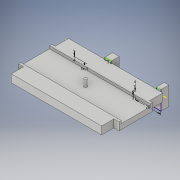
# Autodesk Inventor part: kotelon yläosa
Saved by Autodesk Inventor 2019 (Build 230136000, 136)
## iProperties
Created: 2018-07-24
Part Number: kotelon yläosa
Material: Generic
Document SubType Name: Modeling
Designer: OMISTAJA
Density: 1 g/cm^3
Appearance: Default
Author: OMISTAJA
## iProperties of the stored document kotelon yläosa_3DPrint.ipt
Created: 2018-07-24
Part Number: kotelon yläosa_3DPrint
Material: Generic
Document SubType Name: Modeling
Designer: OMISTAJA
Density: 1 g/cm^3
Appearance: Default
Author: OMISTAJA
Autodesk Inventor part; units mm, degrees
ref_plane "YZ Plane" through (0, 0, 0) normal (1, 0, 0) x (0, 1, 0)
ref_plane "XZ Plane" through (0, 0, 0) normal (0, 1, 0) x (-1, 0, 0)
ref_plane "XY Plane" through (0, 0, 0) normal (0, 0, 1) x (1, 0, 0)
sketch "Sketch1" plane through (0, 0, 0) normal (0, 1, 0) x (-1, 0, 0)
  line L0 (-36.5556, -23.5) -> (36.5556, -23.5)
  line L1 (35, 22.5) -> (-35, 22.5)
  line L2 (-36.5556, -23.5) -> (35, 22.5) construction
  line L3 (36.5556, -23.5) -> (-35, 22.5) construction
  line L4 (-39, 0) -> (-39, -11)
  line L5 (-39, -11) -> (-39, 11)
  line L6 (39, -11) -> (39, 11)
  line L7 (-39, -11) -> (-39, -13)
  line L8 (-39, -13) -> (-36.5556, -13)
  line L9 (-39, 11) -> (-39, 13)
  line L10 (-39, 13) -> (-35, 13)
  line L11 (39, -11) -> (39, -13)
  line L12 (39, -13) -> (36.5556, -13)
  line L13 (39, 11) -> (39, 13)
  line L14 (39, 13) -> (35, 13)
  line L15 (-30.788, 17.5) -> (31, 17.5)
  line L16 (31, 17.5) -> (31, -18.5)
  line L17 (31, -18.5) -> (-30.788, -18.5)
  line L18 (-30.788, -18.5) -> (-30.788, 17.5)
  line L19 (-30.788, 17.5) -> (31, -18.5) construction
  line L20 (31, 17.5) -> (-30.788, -18.5) construction
  line L21 (36.5556, -23.5) -> (36.5556, -13)
  line L22 (35, 13) -> (35, 22.5)
  line L23 (-35, 22.5) -> (-35, 13)
  line L24 (-36.5556, -13) -> (-36.5556, -23.5)
  circle A0 centre (0, 0) radius 1.25
  dimension "d133" = 2.5
  dimension "d169" = 36
  dimension "d170" = 4
  dimension "d171" = 5
  dimension "d180" = 46
  constraints: 50 end point, 11 perpendicular, 7 parallel, 4 point on line, 3 vertical, 2 horizontal, 1 centre point, 1 coincident
  measures "d133" diameter of A0
  measures "d169" distance between parallel lines of L17 L15
  measures "d170" distance between parallel lines of L22 L16
  measures "d171" distance between parallel lines of L0 L17
  measures "d180" distance between parallel lines of L0 L1
extrude "Extrusion39" add sketch "Sketch1" along normal blind 6 contours L24 L8 L7 L4 L5 L9 L10 L23 L1 L22 L14 L13 L6 L11 L12 L21 L0
extrude "Extrusion40" add sketch "Sketch1" against normal blind 2 contours L15 L16 L17 L18
extrude "Extrusion41" add sketch "Sketch1" along normal blind 6 contours L15 L16 L17 L18
extrude "Extrusion42" add sketch "Sketch1" along normal blind 9 contours A0
sketch "Sketch30" plane through (0, 6, 0) normal (0, 1, 0) x (1, 0, 0)
  line L0 (-39, -11.25) -> (39, -11.25)
  line L1 (39, -11.25) -> (39, 11.25)
  line L2 (39, 11.25) -> (-39, 11.25)
  line L3 (-39, 11.25) -> (-39, -11.25)
  circle A0 centre (0, 0) radius 1.25 projected
  line L4 (-39, -11.25) -> (39, 11.25) construction
  line L5 (39, -11.25) -> (-39, 11.25) construction
  dimension "d142" = 78
  dimension "d143" = 22.5
  constraints: 12 end point, 2 midpoint, 2 parallel, 1 horizontal, 1 perpendicular
  measures "d142" distance of L2.end L1.end
  measures "d143" distance of L1.end L0.end
extrude "Extrusion43" cut sketch "Sketch30" against normal blind 2
sketch "Sketch31" plane through (36.5556, 0, -23.5) normal (0, 0, -1) x (-1, 0, 0)
  line L0 (67.5556, 0) -> (5.7676, 0) projected
  line L1 (67.5556, 0) -> (67.5556, -2) projected
  line L2 (64.95, 0) -> (44.95, 0)
  line L3 (44.95, 0) -> (44.95, 7.5)
  line L4 (39.95, 7.5) -> (39.95, -7)
  line L5 (39.95, -7) -> (58.95, -7)
  line L6 (58.95, -7) -> (58.95, -4)
  line L7 (58.95, -4) -> (44.95, -4)
  line L8 (44.95, -4) -> (44.95, 0)
  line L9 (75.5556, 4) -> (-2.4444, 4) projected
  line L10 (5.05, 0) -> (5.05, 4)
  line L11 (1.5556, 0) -> (1.5556, 6) projected
  line L12 (71.5556, 0) -> (1.5556, 0) projected
  line L13 (1.5556, 0) -> (1.5556, -7)
  line L14 (1.5556, -7) -> (21.5556, -7)
  line L15 (21.5556, -7) -> (21.5556, -4)
  line L16 (21.5556, -4) -> (5.05, -4)
  line L17 (5.7676, 0) -> (5.7676, -2) projected
  line L18 (5.05, -4) -> (5.05, 0)
  line L19 (44.95, 7.5) -> (39.95, 7.5)
  line L20 (5.05, 4) -> (5.05, 7.5)
  line L21 (5.05, 7.5) -> (1.5556, 7.5)
  line L22 (1.5556, 7.5) -> (1.5556, -7)
  point P0 (36.5556, 0)
  point P1 (-2.4444, 4)
  point P2 (66, 0)
  point P3 (4.212, 0)
  dimension "d152" = 5
  dimension "d157" = 20
  dimension "d163" = 4
  dimension "d164" = 4
  dimension "d187" = 3
  dimension "d188" = 3
  constraints: 34 end point, 9 perpendicular, 4 point on line, 2 horizontal, 2 vertical, 1 collinear, 5 other
  measures "d152" distance of L3.end L4.start
  measures "d157" distance of L13.end L14.end
  measures "d163" distance between parallel lines of L16 L0
  measures "d164" distance between parallel lines of L7 L0
  measures "d187" distance between parallel lines of L5 L7
  measures "d188" distance between parallel lines of L14 L16
extrude "Extrusion51" cut sketch "Sketch31" along normal blind 10 contours L18 L16 L15 L14 L13 L12
extrude "Extrusion52" cut sketch "Sketch31" along normal blind 10 contours L12 L11 L9 L10 | L9 L11 L22 L21 L20
extrude "Extrusion54" add sketch "Sketch31" along normal blind 6 contours L12 L11 L9 L10 | L18 L16 L15 L14 L13 L12 | L9 L11 L22 L21 L20
extrude "Extrusion55" add sketch "Sketch31" along normal blind 6 contours L8 L7 L6 L5 L4 L0 | L0 L4 L9 L3 | L9 L4 L19 L3
equation "\"d187\" = d188"
body "Solid3"
